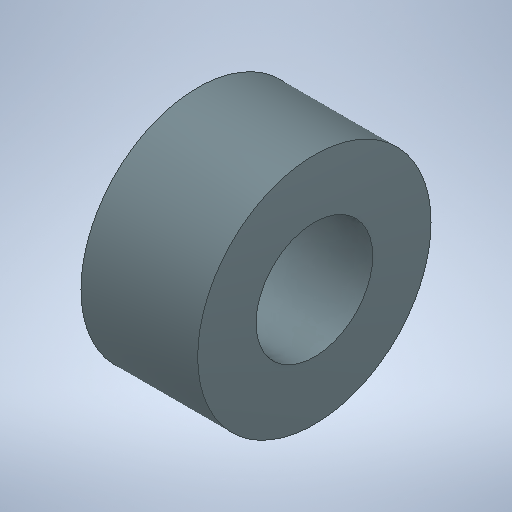
# Autodesk Inventor part: 204 part 1
Saved by Autodesk Inventor 2025.1 (Build 291241000, 241)
## iProperties
Created: 2024-09-02
Part Number: 204 part 1
Material: Lead
Document SubType Name: Modeling
Designer: ffogue
Density: 11.34 g/cm^3
Appearance: Lead
Author: ffogue
Autodesk Inventor part; units mm, degrees
ref_plane "YZ Plane" through (0, 0, 0) normal (1, 0, 0) x (0, 1, 0)
ref_plane "XZ Plane" through (0, 0, 0) normal (0, 1, 0) x (-1, 0, 0)
ref_plane "XY Plane" through (0, 0, 0) normal (0, 0, 1) x (1, 0, 0)
sketch "Sketch1" plane through (0, 0, 0) normal (0, 0, 1) x (1, 0, 0)
  line L0 (0.0275, 3) -> (0.0275, 6)
  line L1 (0.0275, 6) -> (6.0275, 6)
  line L2 (6.0275, 6) -> (6.0275, 3)
  line L3 (6.0275, 3) -> (0.0275, 3)
  line L4 (0, 0) -> (6.0275, 0)
  dimension "d0" = 6
  dimension "d1" = 12
  dimension "d2" = 6
  constraints: 10 end point, 2 perpendicular, 1 horizontal, 1 parallel, 1 vertical, 1 vertical alignment
  measures "d0" diameter of L3 L4
  measures "d1" diameter of L1 L4
  measures "d2" distance of L0.end L1.end
revolve "Revolution1" add sketch "Sketch1" angle 360 about axis through (0, 0, 0) along (1, 0, 0)
body "Solid1"
